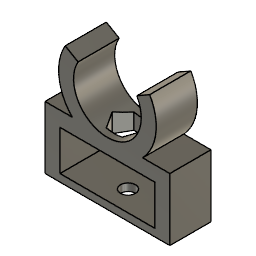
Pump mount (Autodesk Fusion 360 design; units mm, degrees)
part number: 2025-11-16-12-28-37-608
Autodesk Fusion 360 part; units mm, degrees
sketch "Sketch10" plane through (0, 0, 0) normal (0, 1, 0) x (1, 0, 0)
  circle A0 centre (0, 0) radius 13.55
  circle A1 centre (0, 0) radius 19.55
  dimension "d15" = 27.1
  dimension "d16" = 6
  constraint coincident A0.centre A1.centre
  measures "d15" diameter of A0
  measures "d16" distance of A0 A1
extrude "Extrude5" add sketch "Sketch10" along normal blind 16.5
sketch "Sketch11" plane through (0, 16.5, 0) normal (0, 1, 0) x (-1, 0, 0)
  circle A0 centre (0, 0) radius 13.55
  circle A1 centre (0, 0) radius 19.55
  line L0 (0, 0) -> (19.55, 0) construction
  line L1 (0, 0) -> (16.9308, 9.775)
  line L2 (0, 0) -> (0, 19.55) construction
  line L3 (0, 0) -> (-16.9308, 9.775)
  dimension "d19" = 30
  constraint coincident A0.centre A1.centre
  constraint coincident A1 L0.end
  constraint horizontal L0
  constraint coincident A1 L1.end
  constraint coincident A1 L2.end
  constraint vertical L2
  constraint symmetric A0.centre L2 A1.centre
  constraint symmetric L1.end L2 L3.end
  measures "d19" angle of L0 L1
extrude "Extrude6" cut sketch "Sketch11" against normal up to surface (16.5 mm away) contours A0 A1 L1 L3 picked at (-14.6501, 9.5797)
sketch "Sketch13" plane through (0, 0, 0) normal (0, -1, 0) x (1, 0, 0)
  line L0 (-11.7346, 6.775) -> (-16.9308, 9.775)
  arc A0 (-16.9308, 9.775) -> (16.9308, 9.775) centre (0, 0) ccw
  line L1 (16.9308, 9.775) -> (11.7346, 6.775)
  arc A1 (-11.7346, 6.775) -> (11.7346, 6.775) centre (0, 0) ccw
  line L2 (-25, -13.55) -> (25, -13.55)
  line L3 (25, -13.55) -> (25, -38.55)
  line L4 (25, -38.55) -> (-25, -38.55)
  line L5 (-25, -38.55) -> (-25, -13.55)
  line L6 (-19, -19.55) -> (19, -19.55)
  line L7 (19, -19.55) -> (19, -35.55)
  line L8 (19, -35.55) -> (-19, -35.55)
  line L9 (-19, -35.55) -> (-19, -19.55)
  line L10 (0, -13.55) -> (0, -38.55) construction
  point P0 (0, -13.55)
  point P1 (0, -19.55)
  dimension "d25" = 6
  dimension "d26" = 3
  dimension "d27" = 6
  dimension "d28" = 6
  dimension "d30" = 16
  dimension "d31" = 50
  constraint horizontal L2
  constraint vertical L3
  constraint horizontal L4
  constraint vertical L5
  constraint midpoint A1 P0
  constraint midpoint A0 P1
  constraint coincident L2 P0
  constraint horizontal L6
  constraint vertical L7
  constraint horizontal L8
  constraint vertical L9
  constraint coincident P0 L10.start
  constraint midpoint L4 L10.end
  constraint perpendicular L4 L10
  measures "d25" distance of L2 L6
  measures "d26" distance of L4 L8
  measures "d27" distance of L5 L9
  measures "d28" distance of L3 L7
  measures "d30" distance of L6 L8
  measures "d31" distance of L3 L5
extrude "Extrude8" add sketch "Sketch13" against normal up to surface (16.5 mm away) contours A0 L2 L3 L4 L5
sketch "Sketch14" plane through (0, 0, -38.55) normal (0, 0, -1) x (1, 0, 0)
  line L0 (-25, -16.5) -> (25, -16.5)
  line L1 (25, -16.5) -> (25, 0)
  line L2 (25, 0) -> (-25, 0)
  line L3 (-25, 0) -> (-25, -16.5)
  line L4 (6.3509, -8.25) -> (3.1754, -2.75)
  line L5 (3.1754, -2.75) -> (-3.1754, -2.75)
  line L6 (-3.1754, -2.75) -> (-6.3509, -8.25)
  line L7 (-6.3509, -8.25) -> (-3.1754, -13.75)
  line L8 (-3.1754, -13.75) -> (3.1754, -13.75)
  line L9 (3.1754, -13.75) -> (6.3509, -8.25)
  line L10 (-25, -8.25) -> (25, -8.25) construction
  line L11 (0, 0) -> (0, -16.5) construction
  point P0 (0, -8.25)
  dimension "d34" = 11
  constraint midpoint L3 L10.start
  constraint midpoint L1 L10.end
  constraint coincident P0 L10
  constraint coincident L11.start origin
  constraint midpoint L0 L11.end
  constraint coincident P0 L11
  constraint coincident L6.end L10
  measures "d34" distance of L5 L8
extrude "Extrude9" cut sketch "Sketch14" along normal up to surface from surface at -4 contours L4 L5 L6 L7 L8 L9 end surface at (13.0436, 11, 3.6699)
sketch "Sketch15" plane through (0, 0, -38.55) normal (0, 0, -1) x (1, 0, 0)
  line L0 (-25, -16.5) -> (25, -16.5)
  line L1 (25, -16.5) -> (25, 0)
  line L2 (25, 0) -> (-25, 0)
  line L3 (-25, 0) -> (-25, -16.5)
  circle A0 centre (0, -8.25) radius 3
  line L4 (0, 0) -> (0, -16.5) construction
  line L5 (-25, -8.25) -> (25, -8.25) construction
  dimension "d38" = 6
  constraint coincident L4.start origin
  constraint midpoint L0 L4.end
  constraint midpoint L3 L5.start
  constraint midpoint L1 L5.end
  constraint coincident A0.centre L5
  constraint coincident A0.centre L4
  measures "d38" diameter of A0
extrude "Extrude10" cut sketch "Sketch15" against normal up to surface (3 mm away) contours A0
extrude "Extrude7" [suppressed]
extrude "Extrude2" [suppressed]
sketch "Sketch3" plane through (0, 17.78, 0) normal (0, 1, 0) x (-1, 0, 0)
  circle A0 centre (0, 0) radius 15.875
  arc A1 (15.5543, -15.875) -> (-15.5543, -15.875) centre (0, 0) ccw
  line L0 (-15.5543, -15.875) -> (-38.1, -15.875)
  line L1 (-38.1, -15.875) -> (-38.1, -22.225)
  line L2 (-38.1, -22.225) -> (38.1, -22.225)
  line L3 (38.1, -22.225) -> (38.1, -15.875)
  line L4 (38.1, -15.875) -> (15.5543, -15.875)
  line L5 (-33.6611, 21.024) -> (-33.02, 21.024) construction
  constraint horizontal L5
equation "d17 = ( 33 / 2 ) * 1 mm"
